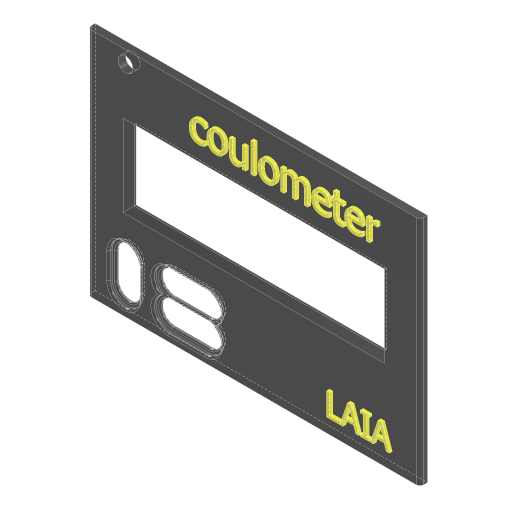
# Autodesk Inventor part: molduraPainel3
Saved by Autodesk Inventor 2023 (Build 270158000, 158)
## iProperties
Created: 2023-09-15
Part Number: molduraPainel3
Material: Generic
Document SubType Name: Modeling
Designer: Claudimir
Density: 1 g/cm^3
Appearance: Default
Author: Claudimir
Autodesk Inventor part; units mm, degrees
ref_plane "YZ Plane" through (0, 0, 0) normal (1, 0, 0) x (0, 1, 0)
ref_plane "XZ Plane" through (0, 0, 0) normal (0, 1, 0) x (-1, 0, 0)
ref_plane "XY Plane" through (0, 0, 0) normal (0, 0, 1) x (1, 0, 0)
sketch "Sketch1" plane through (0, 0, 0) normal (0, 0, 1) x (1, 0, 0)
  line L0 (-41, -18) -> (39, -18) construction
  line L1 (40, -18) -> (40, 18) construction
  line L2 (40, 18) -> (-40, 18) construction
  line L3 (-40, 18) -> (-40, -18) construction
  line L4 (-37.5, -15.5) -> (37.5, -15.5) construction
  line L5 (37.5, -15.5) -> (37.5, 15.5) construction
  line L6 (37.5, 15.5) -> (-37.5, 15.5) construction
  line L7 (-37.5, 15.5) -> (-37.5, -15.5) construction
  line L8 (-40, -18) -> (40, -18) construction
  line L9 (-40, 18) -> (40, 18) construction
  line L10 (-35.9, -12) -> (35.9, -12) construction
  line L11 (35.9, -12) -> (35.9, 11.7) construction
  line L12 (35.9, 11.7) -> (-35.9, 11.7) construction
  line L13 (-35.9, 11.7) -> (-35.9, -12) construction
  line L14 (-40, -18) -> (40, -18) construction
  line L15 (40, -18) -> (40, -32.5) construction
  line L16 (40, -32.5) -> (-40, -32.5) construction
  line L17 (-40, -32.5) -> (-40, -18) construction
  line L18 (-40, 18) -> (40, 18) construction
  line L19 (40, 18) -> (40, 25.5) construction
  line L20 (40, 25.5) -> (-40, 25.5) construction
  line L21 (-40, 25.5) -> (-40, 18) construction
  line L22 (-40, -32.5) -> (-34.8, -32.5) construction
  line L23 (-34.8, -32.5) -> (-34.8, -27.3) construction
  line L24 (-34.8, -27.3) -> (-40, -27.3) construction
  line L25 (-40, -27.3) -> (-40, -32.5) construction
  line L26 (-40, -32.5) -> (-17, -32.5) construction
  line L27 (-17, -32.5) -> (-17, -29.1) construction
  line L28 (-40, -29.1) -> (-40, -32.5) construction
  line L29 (-18, -29.1) -> (-18, -22.1) construction
  circle A0 centre (-34.8, -27.3) radius 1.7 construction
  circle A1 centre (-18, -22.1) radius 1.7 construction
  circle A2 centre (-18, -29.1) radius 1.7 construction
  line L30 (-23, -22.1) -> (-13, -22.1) construction
  line L31 (-23, -24.6) -> (-13, -24.6) construction
  line L32 (-13, -19.6) -> (-23, -19.6) construction
  arc A3 (-23, -19.6) -> (-23, -24.6) centre (-23, -22.1) ccw construction
  arc A4 (-13, -24.6) -> (-13, -19.6) centre (-13, -22.1) ccw construction
  line L33 (-23, -29.1) -> (-13, -29.1) construction
  line L34 (-23, -31.6) -> (-13, -31.6) construction
  line L35 (-13, -26.6) -> (-23, -26.6) construction
  arc A5 (-23, -26.6) -> (-23, -31.6) centre (-23, -29.1) ccw construction
  arc A6 (-13, -31.6) -> (-13, -26.6) centre (-13, -29.1) ccw construction
  line L36 (-34.8, -22.1) -> (-34.8, -29.1) construction
  line L37 (-18, -29.1) -> (-18, -22.1) construction
  line L38 (-34.8, -29.1) -> (-34.8, -22.1) construction
  line L39 (-32.3, -29.1) -> (-32.3, -22.1) construction
  line L40 (-37.3, -22.1) -> (-37.3, -29.1) construction
  arc A7 (-37.3, -29.1) -> (-32.3, -29.1) centre (-34.8, -29.1) ccw construction
  arc A8 (-32.3, -22.1) -> (-37.3, -22.1) centre (-34.8, -22.1) ccw construction
  line L41 (-28, -25.6) -> (-8, -25.6) construction
  line L42 (-10.5, -22.1) -> (-25.5, -22.1) construction
  line L43 (-25.5, -29.1) -> (-10.5, -29.1) construction
  line L44 (-41.5, 27) -> (-41.5, -35)
  line L45 (-41.5, -35) -> (41.5, -35)
  line L46 (41.5, -35) -> (41.5, 27)
  line L47 (41.5, 27) -> (-41.5, 27)
  line L48 (-31.7, -22.1) -> (-31.7, -29.1)
  arc A9 (-37.9, -29.1) -> (-31.7, -29.1) centre (-34.8, -29.1) ccw
  line L49 (-37.9, -29.1) -> (-37.9, -22.1)
  arc A10 (-31.7, -22.1) -> (-37.9, -22.1) centre (-34.8, -22.1) ccw
  line L50 (-23, -19) -> (-13, -19)
  arc A11 (-13, -25.2) -> (-13, -19) centre (-13, -22.1) ccw
  line L51 (-13, -25.2) -> (-23, -25.2)
  arc A12 (-23, -19) -> (-23, -25.2) centre (-23, -22.1) ccw
  line L52 (-23, -32.2) -> (-13, -32.2)
  arc A13 (-13, -32.2) -> (-13, -26) centre (-13, -29.1) ccw
  line L53 (-13, -26) -> (-23, -26)
  arc A14 (-23, -26) -> (-23, -32.2) centre (-23, -29.1) ccw
  line L54 (-35.46, 24.66) -> (-33.26, 24.66) construction
  line L55 (-33.26, 24.66) -> (-33.26, 22.46) construction
  line L56 (-33.26, 22.46) -> (-35.46, 22.46) construction
  line L57 (-35.46, 22.46) -> (-35.46, 24.66) construction
  circle A15 centre (-34.36, 23.56) radius 1.1 construction
  circle A16 centre (-34.36, 23.56) radius 2
  line L58 (33.5, -9.6) -> (-33.5, -9.6)
  line L59 (-33.5, -9.6) -> (-33.5, 9.3)
  line L60 (-33.5, 9.3) -> (33.5, 9.3)
  line L61 (33.5, 9.3) -> (33.5, -9.6)
  line L62 (-41.5, 27) -> (-44.5, 27)
  line L63 (-44.5, 27) -> (-44.5, -35)
  line L64 (-44.5, -35) -> (-41.5, -35)
  line L65 (-41.5, -35) -> (-41.5, 27)
  line L66 (41.5, 27) -> (44.5, 27)
  line L67 (44.5, 27) -> (44.5, -35)
  line L68 (44.5, -35) -> (41.5, -35)
  line L69 (41.5, -35) -> (41.5, 27)
  line L70 (-36.3, 25.5) -> (-26.3, 25.5) construction
  line L71 (-26.3, 25.5) -> (-26.3, 20.5) construction
  line L72 (-26.3, 20.5) -> (-36.3, 20.5) construction
  line L73 (-36.3, 20.5) -> (-36.3, 25.5) construction
  line L74 (-36.3, 25.5) -> (-34.1, 25.5) construction
  line L75 (-34.1, 25.5) -> (-34.1, 23.3) construction
  line L76 (-34.1, 23.3) -> (-36.3, 23.3) construction
  line L77 (-36.3, 23.3) -> (-36.3, 25.5) construction
  line L78 (-25.8, 20) -> (-25.8, 26) construction
  line L79 (-25.8, 26) -> (-36.8, 26) construction
  line L80 (-36.8, 26) -> (-36.8, 20) construction
  line L81 (-36.8, 20) -> (-25.8, 20) construction
  line L82 (-36.8, 26) -> (-34.36, 26) construction
  line L83 (-34.36, 26) -> (-34.36, 23.56) construction
  line L84 (-34.36, 23.56) -> (-36.8, 23.56) construction
  line L85 (-36.8, 23.56) -> (-36.8, 26) construction
  point P0 (0, 0)
  point P1 (-34.8, -25.6)
  point P2 (-18, -25.6)
  dimension "d0" = 80
  dimension "d1" = 36
  dimension "d2" = 75
  dimension "d3" = 31
  dimension "d15" = 5.2
  dimension "d16" = 22
  dimension "d17" = 3.4
  dimension "d18" = 7
  dimension "d19" = 3.4
  dimension "d20" = 3.4
  dimension "d21" = 3.4
  dimension "d43" = 5
  dimension "d44" = 5
  dimension "d46" = 5
  dimension "d51" = 7
  dimension "d52" = 5
  dimension "d70" = 83
  dimension "d82" = 0.6
  dimension "d83" = 0.6
  dimension "d84" = 0.6
  dimension "d87" = 2.2
  dimension "d88" = 2.2
  dimension "d89" = 4
  dimension "d92" = 2.4
  dimension "d102" = 3
  dimension "d103" = 3
  dimension "d107" = 2.2
  dimension "d108" = 2.2
  dimension "d109" = 0.5
  dimension "d110" = 2.44
  dimension "d111" = 2.44
  constraints: 180 end point, 40 equal length, 28 point on circle, 18 horizontal, 17 centre point, 15 perpendicular, 15 tangent, 5 coincident, 3 midpoint, 3 point on line, 1 vertical, 18 other
  measures "d0" distance of L2.end L1.end
  measures "d1" distance of L1.start L1.end
  measures "d2" distance of L6.end L5.end
  measures "d3" distance of L5.end L4.end
  measures "d15" distance of L23.end L22.end
  measures "d16" distance of L28.start L29.start
  measures "d17" distance of L27.end L26.end
  measures "d18" distance of L29.start L29.end
  measures "d19" diameter of A0
  measures "d20" diameter of A1
  measures "d21" diameter of A2
  measures "d43" distance of L37.end L30.end
  measures "d44" diameter of A4
  measures "d46" diameter of A6
  measures "d51" distance of L36.end L36.start
  measures "d52" diameter of A8
  measures "d70" distance of L45.end L44.end
  measures "d82" distance between parallel lines of L39 L48
  measures "d83" distance between parallel lines of L32 L50
  measures "d84" radial gap between concentric circles of A5 A14
  measures "d87" distance of L56.start L56.end
  measures "d88" distance of L54.end L56.start
  measures "d89" diameter of A16
  measures "d92" distance between parallel lines of L10 L58
  measures "d102" distance of L64.end L63.end
  measures "d103" distance of L67.end L68.end
  measures "d107" distance of L76.start L76.end
  measures "d108" distance of L74.end L76.start
  measures "d109" distance between parallel lines of L71 L78
  measures "d110" distance of L83.end L84.end
  measures "d111" distance of L82.end L83.end
extrude "corpo" add sketch "Sketch1" along normal blind 2 contours L47 L46 L45 L44 | A16 | L58 L59 L60 L61
extrude "furo" cut sketch "Sketch1" along normal blind 2 contours A16
extrude "Extrusion11" cut sketch "Sketch1" along normal through all contours L58 L59 L60 L61
chamfer "Chamfer1" distance 1.5 angle 45 4 edges at (-33.5, -0.15, 2) (0, 9.3, 2) (0, -9.6, 2) (33.5, -0.15, 2)
fillet "Fillet2" radius 0.4 12 edges at (-18, -19, 0) (-9.9, -22.1, 0) (-18, -25.2, 0) (-26.1, -22.1, 0) (-18, -26, 0) (-9.9, -29.1, 0) (-18, -32.2, 0) (-26.1, -29.1, 0) (-31.7, -25.6, 0) (-34.8, -32.2, 0) (-37.9, -25.6, 0) (-34.8, -19, 0)
sketch "Sketch3" plane through (0, 0, 2) normal (0, 0, 1) x (1, 0, 0)
  line L0 (-21.3139, 23.4826) -> (37.1514, 23.4826) construction
  line L1 (37.1514, 23.4826) -> (37.1514, -33.0376) construction
  line L2 (37.1514, -33.0376) -> (-21.3139, -33.0376) construction
  line L3 (-21.3139, -33.0376) -> (-21.3139, 23.4826) construction
  spline S0 degree 2 poles (-13.896, 15.5207) (-14.4795, 15.5207) (-15.4458, 15.8793) (-15.7923, 16.2439) knots 0 0 0 1 2 2 2
  spline S1 degree 2 poles (-15.7923, 16.2439) (-16.1387, 16.6025) (-16.5216, 17.7087) (-16.5216, 18.4502) knots 0 0 0 1 2 2 2
  spline S2 degree 2 poles (-16.5216, 18.4502) (-16.5216, 19.1917) (-16.1266, 20.2735) (-15.7923, 20.6382) knots 0 0 0 1 2 2 2
  spline S3 degree 2 poles (-15.7923, 20.6382) (-15.458, 21.0089) (-14.4673, 21.404) (-13.896, 21.404) knots 0 0 0 1 2 2 2
  spline S4 degree 2 poles (-13.896, 21.404) (-13.4341, 21.404) (-12.571, 21.1426) (-12.2368, 20.9725) knots 0 0 0 1 2 2 2
  line L4 (-12.2368, 20.9725) -> (-12.2368, 19.9088)
  line L5 (-12.2368, 19.9088) -> (-12.2915, 19.9088)
  spline S5 degree 2 poles (-12.2915, 19.9088) (-12.3948, 19.9939) (-12.7108, 20.2127) (-12.9357, 20.3282) knots 0 0 0 1 2 2 2
  spline S6 degree 2 poles (-12.9357, 20.3282) (-13.1363, 20.4255) (-13.6711, 20.5774) (-13.9142, 20.5774) knots 0 0 0 1 2 2 2
  spline S7 degree 2 poles (-13.9142, 20.5774) (-14.6497, 20.5774) (-15.5431, 19.4652) (-15.5431, 18.4502) knots 0 0 0 1 2 2 2
  spline S8 degree 2 poles (-15.5431, 18.4502) (-15.5431, 17.4595) (-14.68, 16.3473) (-13.9142, 16.3473) knots 0 0 0 1 2 2 2
  spline S9 degree 2 poles (-13.9142, 16.3473) (-13.4523, 16.3473) (-12.6136, 16.7302) (-12.2915, 17.028) knots 0 0 0 1 2 2 2
  line L6 (-12.2915, 17.028) -> (-12.2368, 17.028)
  line L7 (-12.2368, 17.028) -> (-12.2368, 15.9644)
  spline S10 degree 2 poles (-12.2368, 15.9644) (-12.3766, 15.8975) (-12.802, 15.7091) (-12.9722, 15.6665) knots 0 0 0 1 2 2 2
  spline S11 degree 2 poles (-12.9722, 15.6665) (-13.2153, 15.5936) (-13.5982, 15.5207) (-13.896, 15.5207) knots 0 0 0 1 2 2 2
  spline S12 degree 2 poles (-6.7485, 18.4623) (-6.7485, 17.0401) (-8.116, 15.4903) (-9.2586, 15.4903) knots 0 0 0 1 2 2 2
  spline S13 degree 2 poles (-9.2586, 15.4903) (-10.4317, 15.4903) (-11.7749, 17.0888) (-11.7749, 18.4623) knots 0 0 0 1 2 2 2
  spline S14 degree 2 poles (-11.7749, 18.4623) (-11.7749, 19.8724) (-10.3891, 21.4344) (-9.2586, 21.4344) knots 0 0 0 1 2 2 2
  spline S15 degree 2 poles (-9.2586, 21.4344) (-8.116, 21.4344) (-6.7485, 19.8785) (-6.7485, 18.4623) knots 0 0 0 1 2 2 2
  spline S16 degree 2 poles (-7.727, 18.4623) (-7.727, 19.5563) (-8.5232, 20.62) (-9.2586, 20.62) knots 0 0 0 1 2 2 2
  spline S17 degree 2 poles (-9.2586, 20.62) (-9.9941, 20.62) (-10.7963, 19.5563) (-10.7963, 18.4623) knots 0 0 0 1 2 2 2
  spline S18 degree 2 poles (-10.7963, 18.4623) (-10.7963, 17.3987) (-9.9941, 16.3047) (-9.2586, 16.3047) knots 0 0 0 1 2 2 2
  spline S19 degree 2 poles (-9.2586, 16.3047) (-8.5293, 16.3047) (-7.727, 17.3805) (-7.727, 18.4623) knots 0 0 0 1 2 2 2
  line L8 (-1.4001, 15.6483) -> (-2.3482, 15.6483)
  line L9 (-2.3482, 15.6483) -> (-2.3482, 16.2682)
  spline S20 degree 2 poles (-2.3482, 16.2682) (-2.7858, 15.8853) (-3.5698, 15.4903) (-4.0561, 15.4903) knots 0 0 0 1 2 2 2
  spline S21 degree 2 poles (-4.0561, 15.4903) (-4.4207, 15.4903) (-5.071, 15.7334) (-5.3081, 15.9947) knots 0 0 0 1 2 2 2
  spline S22 degree 2 poles (-5.3081, 15.9947) (-5.5512, 16.2561) (-5.8186, 17.0523) (-5.8186, 17.6236) knots 0 0 0 1 2 2 2
  line L10 (-5.8186, 17.6236) -> (-5.8186, 21.2764)
  line L11 (-5.8186, 21.2764) -> (-4.8705, 21.2764)
  line L12 (-4.8705, 21.2764) -> (-4.8705, 18.0673)
  spline S23 degree 2 poles (-4.8705, 18.0673) (-4.8705, 17.6175) (-4.8036, 17.028) (-4.6881, 16.8092) knots 0 0 0 1 2 2 2
  spline S24 degree 2 poles (-4.6881, 16.8092) (-4.5727, 16.5904) (-4.1776, 16.3898) (-3.8069, 16.3898) knots 0 0 0 1 2 2 2
  spline S25 degree 2 poles (-3.8069, 16.3898) (-3.4604, 16.3898) (-2.6764, 16.7849) (-2.3482, 17.0705) knots 0 0 0 1 2 2 2
  line L13 (-2.3482, 17.0705) -> (-2.3482, 21.2764)
  line L14 (-2.3482, 21.2764) -> (-1.4001, 21.2764)
  line L15 (-1.4001, 21.2764) -> (-1.4001, 15.6483)
  line L16 (0.9399, 15.6483) -> (-0.0082, 15.6483)
  line L17 (-0.0082, 15.6483) -> (-0.0082, 23.4826)
  line L18 (-0.0082, 23.4826) -> (0.9399, 23.4826)
  line L19 (0.9399, 23.4826) -> (0.9399, 15.6483)
  spline S26 degree 2 poles (6.9569, 18.4623) (6.9569, 17.0401) (5.5894, 15.4903) (4.4468, 15.4903) knots 0 0 0 1 2 2 2
  spline S27 degree 2 poles (4.4468, 15.4903) (3.2738, 15.4903) (1.9306, 17.0888) (1.9306, 18.4623) knots 0 0 0 1 2 2 2
  spline S28 degree 2 poles (1.9306, 18.4623) (1.9306, 19.8724) (3.3163, 21.4344) (4.4468, 21.4344) knots 0 0 0 1 2 2 2
  spline S29 degree 2 poles (4.4468, 21.4344) (5.5894, 21.4344) (6.9569, 19.8785) (6.9569, 18.4623) knots 0 0 0 1 2 2 2
  spline S30 degree 2 poles (5.9784, 18.4623) (5.9784, 19.5563) (5.1822, 20.62) (4.4468, 20.62) knots 0 0 0 1 2 2 2
  spline S31 degree 2 poles (4.4468, 20.62) (3.7114, 20.62) (2.9091, 19.5563) (2.9091, 18.4623) knots 0 0 0 1 2 2 2
  spline S32 degree 2 poles (2.9091, 18.4623) (2.9091, 17.3987) (3.7114, 16.3047) (4.4468, 16.3047) knots 0 0 0 1 2 2 2
  spline S33 degree 2 poles (4.4468, 16.3047) (5.1761, 16.3047) (5.9784, 17.3805) (5.9784, 18.4623) knots 0 0 0 1 2 2 2
  line L20 (14.311, 15.6483) -> (14.311, 18.906)
  spline S34 degree 2 poles (14.311, 18.906) (14.311, 19.295) (14.2503, 19.9575) (14.153, 20.1398) knots 0 0 0 1 2 2 2
  spline S35 degree 2 poles (14.153, 20.1398) (14.0558, 20.3404) (13.685, 20.5349) (13.3629, 20.5349) knots 0 0 0 1 2 2 2
  spline S36 degree 2 poles (13.3629, 20.5349) (13.0712, 20.5349) (12.4026, 20.1763) (12.0501, 19.8359) knots 0 0 0 1 2 2 2
  spline S37 degree 2 poles (12.0501, 19.8359) (12.0562, 19.7508) (12.0683, 19.5138) (12.0683, 19.3558) knots 0 0 0 1 2 2 2
  line L21 (12.0683, 19.3558) -> (12.0683, 15.6483)
  line L22 (12.0683, 15.6483) -> (11.1202, 15.6483)
  line L23 (11.1202, 15.6483) -> (11.1202, 18.906)
  spline S38 degree 2 poles (11.1202, 18.906) (11.1202, 19.295) (11.0594, 19.9575) (10.9622, 20.1398) knots 0 0 0 1 2 2 2
  spline S39 degree 2 poles (10.9622, 20.1398) (10.8649, 20.3404) (10.4942, 20.5349) (10.1721, 20.5349) knots 0 0 0 1 2 2 2
  spline S40 degree 2 poles (10.1721, 20.5349) (9.8682, 20.5349) (9.1935, 20.152) (8.8775, 19.8541) knots 0 0 0 1 2 2 2
  line L24 (8.8775, 19.8541) -> (8.8775, 15.6483)
  line L25 (8.8775, 15.6483) -> (7.9294, 15.6483)
  line L26 (7.9294, 15.6483) -> (7.9294, 21.2764)
  line L27 (7.9294, 21.2764) -> (8.8775, 21.2764)
  line L28 (8.8775, 21.2764) -> (8.8775, 20.6564)
  spline S41 degree 2 poles (8.8775, 20.6564) (9.2482, 21.0272) (9.9776, 21.4344) (10.4152, 21.4344) knots 0 0 0 1 2 2 2
  spline S42 degree 2 poles (10.4152, 21.4344) (10.9136, 21.4344) (11.6854, 20.9785) (11.886, 20.4619) knots 0 0 0 1 2 2 2
  spline S43 degree 2 poles (11.886, 20.4619) (12.3175, 20.9421) (13.132, 21.4344) (13.606, 21.4344) knots 0 0 0 1 2 2 2
  spline S44 degree 2 poles (13.606, 21.4344) (13.9707, 21.4344) (14.5663, 21.2095) (14.7851, 20.9542) knots 0 0 0 1 2 2 2
  spline S45 degree 2 poles (14.7851, 20.9542) (15.01, 20.699) (15.2592, 19.9332) (15.2592, 19.3558) knots 0 0 0 1 2 2 2
  line L29 (15.2592, 19.3558) -> (15.2592, 15.6483)
  line L30 (15.2592, 15.6483) -> (14.311, 15.6483)
  spline S46 degree 2 poles (19.0335, 15.5207) (17.6842, 15.5207) (16.2012, 17.0341) (16.2012, 18.4319) knots 0 0 0 1 2 2 2
  spline S47 degree 2 poles (16.2012, 18.4319) (16.2012, 19.8055) (17.6417, 21.4344) (18.8025, 21.4344) knots 0 0 0 1 2 2 2
  spline S48 degree 2 poles (18.8025, 21.4344) (19.3252, 21.4344) (20.1336, 21.1305) (20.4314, 20.8084) knots 0 0 0 1 2 2 2
  spline S49 degree 2 poles (20.4314, 20.8084) (20.7353, 20.4862) (21.0574, 19.5563) (21.0574, 18.8817) knots 0 0 0 1 2 2 2
  line L31 (21.0574, 18.8817) -> (21.0574, 18.3651)
  line L32 (21.0574, 18.3651) -> (17.1615, 18.3651)
  spline S50 degree 2 poles (17.1615, 18.3651) (17.1615, 17.3866) (18.1461, 16.3473) (19.0213, 16.3473) knots 0 0 0 1 2 2 2
  spline S51 degree 2 poles (19.0213, 16.3473) (19.3313, 16.3473) (19.933, 16.487) (20.1761, 16.5964) knots 0 0 0 1 2 2 2
  spline S52 degree 2 poles (20.1761, 16.5964) (20.4314, 16.718) (20.7839, 16.9307) (20.8994, 17.028) knots 0 0 0 1 2 2 2
  line L33 (20.8994, 17.028) -> (20.9541, 17.028)
  line L34 (20.9541, 17.028) -> (20.9541, 15.9947)
  spline S53 degree 2 poles (20.9541, 15.9947) (20.79, 15.9279) (20.2916, 15.7334) (20.0971, 15.6787) knots 0 0 0 1 2 2 2
  spline S54 degree 2 poles (20.0971, 15.6787) (19.8236, 15.5997) (19.3738, 15.5207) (19.0335, 15.5207) knots 0 0 0 1 2 2 2
  spline S55 degree 2 poles (20.1336, 19.0883) (20.1214, 19.4712) (19.9634, 20.0304) (19.8114, 20.2188) knots 0 0 0 1 2 2 2
  spline S56 degree 2 poles (19.8114, 20.2188) (19.6473, 20.4315) (19.1307, 20.6564) (18.7478, 20.6564) knots 0 0 0 1 2 2 2
  spline S57 degree 2 poles (18.7478, 20.6564) (18.371, 20.6564) (17.8422, 20.4315) (17.6234, 20.2127) knots 0 0 0 1 2 2 2
  spline S58 degree 2 poles (17.6234, 20.2127) (17.4107, 19.9879) (17.1919, 19.4469) (17.1615, 19.0883) knots 0 0 0 1 2 2 2
  line L35 (17.1615, 19.0883) -> (20.1336, 19.0883)
  spline S59 degree 2 poles (23.7195, 15.5389) (22.9476, 15.5389) (22.0785, 16.4202) (22.0785, 17.3744) knots 0 0 0 1 2 2 2
  line L36 (22.0785, 17.3744) -> (22.0785, 20.4923)
  line L37 (22.0785, 20.4923) -> (21.4403, 20.4923)
  line L38 (21.4403, 20.4923) -> (21.4403, 21.2764)
  line L39 (21.4403, 21.2764) -> (22.0785, 21.2764)
  line L40 (22.0785, 21.2764) -> (22.0785, 22.893)
  line L41 (22.0785, 22.893) -> (23.0266, 22.893)
  line L42 (23.0266, 22.893) -> (23.0266, 21.2764)
  line L43 (23.0266, 21.2764) -> (24.7709, 21.2764)
  line L44 (24.7709, 21.2764) -> (24.7709, 20.4923)
  line L45 (24.7709, 20.4923) -> (23.0266, 20.4923)
  line L46 (23.0266, 20.4923) -> (23.0266, 17.812)
  spline S60 degree 2 poles (23.0266, 17.812) (23.0266, 17.3866) (23.057, 16.9186) (23.1603, 16.718) knots 0 0 0 1 2 2 2
  spline S61 degree 2 poles (23.1603, 16.718) (23.2454, 16.5417) (23.6283, 16.3655) (23.9565, 16.3655) knots 0 0 0 1 2 2 2
  spline S62 degree 2 poles (23.9565, 16.3655) (24.1875, 16.3655) (24.619, 16.5053) (24.7162, 16.5478) knots 0 0 0 1 2 2 2
  line L47 (24.7162, 16.5478) -> (24.7709, 16.5478)
  line L48 (24.7709, 16.5478) -> (24.7709, 15.6969)
  spline S63 degree 2 poles (24.7709, 15.6969) (24.5035, 15.624) (23.9565, 15.5389) (23.7195, 15.5389) knots 0 0 0 1 2 2 2
  spline S64 degree 2 poles (27.9131, 15.5207) (26.5639, 15.5207) (25.0809, 17.0341) (25.0809, 18.4319) knots 0 0 0 1 2 2 2
  spline S65 degree 2 poles (25.0809, 18.4319) (25.0809, 19.8055) (26.5213, 21.4344) (27.6822, 21.4344) knots 0 0 0 1 2 2 2
  spline S66 degree 2 poles (27.6822, 21.4344) (28.2049, 21.4344) (29.0132, 21.1305) (29.311, 20.8084) knots 0 0 0 1 2 2 2
  spline S67 degree 2 poles (29.311, 20.8084) (29.6149, 20.4862) (29.9371, 19.5563) (29.9371, 18.8817) knots 0 0 0 1 2 2 2
  line L49 (29.9371, 18.8817) -> (29.9371, 18.3651)
  line L50 (29.9371, 18.3651) -> (26.0412, 18.3651)
  spline S68 degree 2 poles (26.0412, 18.3651) (26.0412, 17.3866) (27.0258, 16.3473) (27.901, 16.3473) knots 0 0 0 1 2 2 2
  spline S69 degree 2 poles (27.901, 16.3473) (28.211, 16.3473) (28.8127, 16.487) (29.0558, 16.5964) knots 0 0 0 1 2 2 2
  spline S70 degree 2 poles (29.0558, 16.5964) (29.311, 16.718) (29.6636, 16.9307) (29.779, 17.028) knots 0 0 0 1 2 2 2
  line L51 (29.779, 17.028) -> (29.8337, 17.028)
  line L52 (29.8337, 17.028) -> (29.8337, 15.9947)
  spline S71 degree 2 poles (29.8337, 15.9947) (29.6696, 15.9279) (29.1713, 15.7334) (28.9768, 15.6787) knots 0 0 0 1 2 2 2
  spline S72 degree 2 poles (28.9768, 15.6787) (28.7033, 15.5997) (28.2535, 15.5207) (27.9131, 15.5207) knots 0 0 0 1 2 2 2
  spline S73 degree 2 poles (29.0132, 19.0883) (29.0011, 19.4712) (28.8431, 20.0304) (28.6911, 20.2188) knots 0 0 0 1 2 2 2
  spline S74 degree 2 poles (28.6911, 20.2188) (28.527, 20.4315) (28.0104, 20.6564) (27.6275, 20.6564) knots 0 0 0 1 2 2 2
  spline S75 degree 2 poles (27.6275, 20.6564) (27.2507, 20.6564) (26.7219, 20.4315) (26.5031, 20.2127) knots 0 0 0 1 2 2 2
  spline S76 degree 2 poles (26.5031, 20.2127) (26.2904, 19.9879) (26.0716, 19.4469) (26.0412, 19.0883) knots 0 0 0 1 2 2 2
  line L53 (26.0412, 19.0883) -> (29.0132, 19.0883)
  line L54 (33.8815, 20.2614) -> (33.8329, 20.2614)
  spline S77 degree 2 poles (33.8329, 20.2614) (33.7235, 20.2917) (33.4865, 20.3039) (33.3224, 20.3039) knots 0 0 0 1 2 2 2
  spline S78 degree 2 poles (33.3224, 20.3039) (32.9395, 20.3039) (32.1858, 19.9696) (31.8455, 19.6414) knots 0 0 0 1 2 2 2
  line L55 (31.8455, 19.6414) -> (31.8455, 15.6483)
  line L56 (31.8455, 15.6483) -> (30.8973, 15.6483)
  line L57 (30.8973, 15.6483) -> (30.8973, 21.2764)
  line L58 (30.8973, 21.2764) -> (31.8455, 21.2764)
  line L59 (31.8455, 21.2764) -> (31.8455, 20.4376)
  spline S79 degree 2 poles (31.8455, 20.4376) (32.3621, 20.8995) (33.134, 21.2764) (33.4986, 21.2764) knots 0 0 0 1 2 2 2
  spline S80 degree 2 poles (33.4986, 21.2764) (33.6445, 21.2764) (33.7904, 21.2642) (33.8815, 21.246) knots 0 0 0 1 2 2 2
  line L60 (33.8815, 21.246) -> (33.8815, 20.2614)
  line L61 (23.8589, -30.4993) -> (20.3245, -30.4993)
  line L62 (20.3245, -30.4993) -> (20.3245, -24.3993)
  line L63 (20.3245, -24.3993) -> (21.1352, -24.3993)
  line L64 (21.1352, -24.3993) -> (21.1352, -29.7775)
  line L65 (21.1352, -29.7775) -> (23.8589, -29.7775)
  line L66 (23.8589, -29.7775) -> (23.8589, -30.4993)
  line L67 (23.8392, -30.4993) -> (25.8956, -24.3993)
  line L68 (25.8956, -24.3993) -> (26.8941, -24.3993)
  line L69 (26.8941, -24.3993) -> (28.9505, -30.4993)
  line L70 (28.9505, -30.4993) -> (28.0953, -30.4993)
  line L71 (28.0953, -30.4993) -> (27.5417, -28.7938)
  line L72 (27.5417, -28.7938) -> (25.2134, -28.7938)
  line L73 (25.2134, -28.7938) -> (24.6597, -30.4993)
  line L74 (24.6597, -30.4993) -> (23.8392, -30.4993)
  line L75 (27.3192, -28.1018) -> (26.3751, -25.2297)
  line L76 (26.3751, -25.2297) -> (25.4358, -28.1018)
  line L77 (25.4358, -28.1018) -> (27.3192, -28.1018)
  line L78 (31.6545, -30.4993) -> (29.2916, -30.4993)
  line L79 (29.2916, -30.4993) -> (29.2916, -29.8764)
  line L80 (29.2916, -29.8764) -> (30.0677, -29.8764)
  line L81 (30.0677, -29.8764) -> (30.0677, -25.0221)
  line L82 (30.0677, -25.0221) -> (29.2916, -25.0221)
  line L83 (29.2916, -25.0221) -> (29.2916, -24.3993)
  line L84 (29.2916, -24.3993) -> (31.6545, -24.3993)
  line L85 (31.6545, -24.3993) -> (31.6545, -25.0221)
  line L86 (31.6545, -25.0221) -> (30.8784, -25.0221)
  line L87 (30.8784, -25.0221) -> (30.8784, -29.8764)
  line L88 (30.8784, -29.8764) -> (31.6545, -29.8764)
  line L89 (31.6545, -29.8764) -> (31.6545, -30.4993)
  line L90 (32.0005, -30.4993) -> (34.0569, -24.3993)
  line L91 (34.0569, -24.3993) -> (35.0555, -24.3993)
  line L92 (35.0555, -24.3993) -> (37.1119, -30.4993)
  line L93 (37.1119, -30.4993) -> (36.2567, -30.4993)
  line L94 (36.2567, -30.4993) -> (35.703, -28.7938)
  line L95 (35.703, -28.7938) -> (33.3747, -28.7938)
  line L96 (33.3747, -28.7938) -> (32.8211, -30.4993)
  line L97 (32.8211, -30.4993) -> (32.0005, -30.4993)
  line L98 (35.4806, -28.1018) -> (34.5364, -25.2297)
  line L99 (34.5364, -25.2297) -> (33.5972, -28.1018)
  line L100 (33.5972, -28.1018) -> (35.4806, -28.1018)
  point P0 (0, 0)
  constraints: 2 other
extrude "texto" add sketch "Sketch3" along normal blind 0.8 separate body
extrude "Extrusion13" add sketch "Sketch1" along normal up to surface (2 mm away) contours L44 L64 L63 L62 | L66 L67 L68 L46 bodies 1
fillet "Fillet4" radius 1 2 edges at (-44.5, -4, 2) (44.5, -4, 2)
sketch "Sketch4" plane through (0, 0, 2) normal (0, 0, 1) x (1, 0, 0)
  arc A0 (-23, -19) -> (-23, -25.2) centre (-23, -22.1) ccw construction
  arc A1 (-13, -25.6) -> (-13, -18.6) centre (-13, -22.1) ccw construction
  line L0 (-23, -22.1) -> (-13, -22.1) construction
  line L1 (-23, -19) -> (-13, -19) construction
  line L2 (-13, -25.2) -> (-23, -25.2) construction
  arc A2 (-23, -19) -> (-23, -25.2) centre (-23, -22.1) ccw construction
  arc A3 (-13, -25.2) -> (-13, -19) centre (-13, -22.1) ccw construction
  arc A4 (-23, -26) -> (-23, -32.2) centre (-23, -29.1) ccw construction
  arc A5 (-13, -32.2) -> (-13, -26) centre (-13, -29.1) ccw construction
  line L3 (-23, -29.1) -> (-13, -29.1) construction
  line L4 (-23, -26) -> (-13, -26) construction
  line L5 (-13, -32.2) -> (-23, -32.2) construction
  arc A6 (-23, -26) -> (-23, -32.2) centre (-23, -29.1) ccw construction
  arc A7 (-13, -32.2) -> (-13, -26) centre (-13, -29.1) ccw construction
  arc A8 (-31.7, -22.1) -> (-37.9, -22.1) centre (-34.8, -22.1) ccw construction
  arc A9 (-38.3, -29.1) -> (-31.3, -29.1) centre (-34.8, -29.1) ccw construction
  line L6 (-34.8, -22.1) -> (-34.8, -29.1) construction
  line L7 (-37.9, -22.1) -> (-37.9, -29.1) construction
  line L8 (-31.7, -29.1) -> (-31.7, -22.1) construction
  arc A10 (-31.7, -22.1) -> (-37.9, -22.1) centre (-34.8, -22.1) ccw construction
  arc A11 (-37.9, -29.1) -> (-31.7, -29.1) centre (-34.8, -29.1) ccw construction
  line L9 (-13, -18) -> (-23, -18)
  arc A12 (-23, -18) -> (-23, -26.2) centre (-23, -22.1) ccw
  line L10 (-23, -26.2) -> (-13, -26.2)
  arc A13 (-13, -26.2) -> (-13, -18) centre (-13, -22.1) ccw
  line L11 (-23, -33.2) -> (-13, -33.2)
  arc A14 (-13, -33.2) -> (-13, -25) centre (-13, -29.1) ccw
  line L12 (-13, -25) -> (-23, -25)
  arc A15 (-23, -25) -> (-23, -33.2) centre (-23, -29.1) ccw
  line L13 (-30.7, -22.1) -> (-30.7, -29.1)
  arc A16 (-38.9, -29.1) -> (-30.7, -29.1) centre (-34.8, -29.1) ccw
  line L14 (-38.9, -29.1) -> (-38.9, -22.1)
  arc A17 (-30.7, -22.1) -> (-38.9, -22.1) centre (-34.8, -22.1) ccw
  point P0 (0, 0)
  point P1 (-18, -22.1)
  point P2 (-18, -29.1)
  point P3 (-34.8, -25.6)
  point P4 (-25.1354, -25.6)
  point P5 (-10.8646, -25.6)
  dimension "d112" = 1
  dimension "d113" = 1
  dimension "d114" = 1
  constraints: 36 end point, 24 point on circle, 12 centre point, 12 tangent, 7 parallel, 3 midpoint, 1 perpendicular, 9 other
  measures "d112" distance between parallel lines of L1 L9
  measures "d113" radial gap between concentric circles of A6 A15
  measures "d114" distance between parallel lines of L8 L13
extrude "Extrusion14" cut sketch "Sketch4" against normal blind 1 bodies 1
fillet "Fillet5" radius 0.4 12 edges at (-34.8, -32.2, 1) (-31.7, -25.6, 1) (-34.8, -19, 1) (-37.9, -25.6, 1) (-18, -25.2, 1) (-9.9, -22.1, 1) (-18, -19, 1) (-26.1, -22.1, 1) (-18, -32.2, 1) (-9.9, -29.1, 1) (-18, -26, 1) (-26.1, -29.1, 1)
fillet "Fillet6" radius 0.5 10 edges at (-30.7, -25.6, 2) (-34.8, -33.2, 2) (-38.9, -25.6, 2) (-34.8, -18, 2) (-18, -18, 2) (-9.0528, -20.9909, 2) (-26.9472, -20.9909, 2) (-18, -33.2, 2) (-9.0528, -30.2091, 2) (-26.9472, -30.2091, 2)
